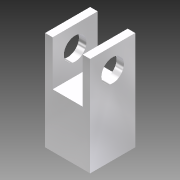
# Autodesk Inventor part: 1in Actuator Clovis 1764
Saved by Autodesk Inventor 2011 (Build 150239000, 239)
## iProperties
Created: 2010-02-13
Part Number: 1in Actuator Clovis 1764
Document SubType Name: Modeling
Designer: jgehrig
Density: 1 g/cm^3
Author: jgehrig
Autodesk Inventor part; units mm, degrees
ref_plane "YZ Plane" through (0, 0, 0) normal (1, 0, 0) x (0, 1, 0)
ref_plane "XZ Plane" through (0, 0, 0) normal (0, 1, 0) x (-1, 0, 0)
ref_plane "XY Plane" through (0, 0, 0) normal (0, 0, 1) x (1, 0, 0)
sketch "Sketch1" plane through (0, 0, 0) normal (0, 0, 1) x (1, 0, 0)
  line L0 (-21.1557, 36.079) -> (-21.1557, -5.831)
  line L1 (-21.1557, -5.831) -> (-2.1057, -5.831)
  line L2 (-2.1057, -5.831) -> (-2.1057, 36.079)
  line L3 (-2.1057, 36.079) -> (-5.2807, 36.079)
  line L4 (-5.2807, 36.079) -> (-5.2807, 17.029)
  line L5 (-5.2807, 17.029) -> (-17.9807, 17.029)
  line L6 (-17.9807, 17.029) -> (-17.9807, 36.079)
  line L7 (-17.9807, 36.079) -> (-21.1557, 36.079)
  point P0 (0, 0)
  dimension "d0" = 19.05
  dimension "d1" = 12.7
  dimension "d2" = 3.175
  dimension "d3" = 3.175
  dimension "d4" = 41.91
  dimension "d5" = 19.05
  dimension "d6" = 0
  constraints: 16 end point, 6 parallel, 1 perpendicular, 1 vertical
  measures "d0" distance of L0.end L1.end
  measures "d1" distance of L4.end L5.end
  measures "d2" distance of L6.end L0.start
  measures "d3" distance of L2.end L3.end
  measures "d4" distance of L0.start L0.end
  measures "d5" distance of L3.end L4.end
  measures "d6" distance between parallel lines of L3 L7
extrude "Extrusion1" add sketch "Sketch1" along normal blind 19.05
sketch "Sketch2" plane through (-21.1557, -5.831, 0) normal (0, -1, 0) x (1, 0, 0)
  circle A0 centre (9.525, 9.525) radius 6.35
  point P0 (21.1557, 0)
  dimension "d9" = 12.7
  constraints: 1 centre point
  measures "d9" diameter of A0
extrude "Extrusion2" cut sketch "Sketch2" against normal blind 21.59
sketch "Sketch3" plane through (-21.1557, -5.831, 0) normal (-1, 0, 0) x (0, 0, 1)
  line L0 (0, 41.91) -> (19.05, 41.91) projected
  circle A0 centre (9.525, 33.02) radius 4.7625
  point P0 (0, 5.831)
  dimension "d12" = 9.525
  dimension "d13" = 8.89
  constraints: 1 centre point
  measures "d12" diameter of A0
  measures "d13" distance from line of L0 A0.centre
extrude "Extrusion3" cut sketch "Sketch3" against normal through all
thread "Thread1" size "1/2-13 UNC" class "2B" standard "ANSI Unified Screw Threads" full length
body "Solid1"
